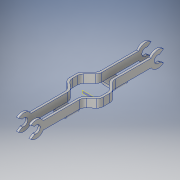
# Autodesk Inventor part: rocker
Saved by Autodesk Inventor 2018 (Build 220112000, 112)
## iProperties
Created: 2018-02-27
Part Number: rocker
Material: Aluminum 6061
Document SubType Name: Modeling
Designer: 238438
Density: 2.7 g/cm^3
Appearance: Aluminum - Flat
Author: 238438
Autodesk Inventor part; units mm, degrees
ref_plane "YZ Plane" through (0, 0, 0) normal (1, 0, 0) x (0, 1, 0)
ref_plane "XZ Plane" through (0, 0, 0) normal (0, 1, 0) x (-1, 0, 0)
ref_plane "XY Plane" through (0, 0, 0) normal (0, 0, 1) x (1, 0, 0)
sketch "Sketch1" plane through (0, 0, 0) normal (0, 1, 0) x (-1, 0, 0)
  line L0 (-1.778, -22.923) -> (-1.778, 0)
  line L1 (-0.508, -7.6359) -> (-0.508, -7.8464)
  line L2 (0, -7.62) -> (2.3608, -9.743)
  line L3 (-0.508, -7.8464) -> (1.8528, -9.9694)
  line L4 (2.3608, -10.0755) -> (2.3608, -9.743)
  line L5 (1.8528, -9.9694) -> (1.8528, -12.5094)
  line L6 (2.3608, -12.7283) -> (2.3608, -10.0755)
  line L7 (1.8528, -12.5094) -> (-0.508, -14.8702)
  line L8 (2.3608, -12.7283) -> (0, -15.1057)
  line L9 (-0.508, -15.1057) -> (-0.508, -25.2657)
  line L10 (-0.508, -25.2657) -> (0, -25.2657)
  line L11 (0, -25.2657) -> (0, -15.1057)
  line L12 (-0.508, -15.1057) -> (-0.508, -14.8702)
  line L13 (-0.508, -7.6359) -> (-0.508, 2.5241)
  line L14 (-0.508, 2.5241) -> (0, 2.5241)
  line L15 (0, 2.5241) -> (0, -7.62)
  line L16 (-5.4088, -9.9694) -> (-5.4088, -12.5094)
  line L17 (-5.9168, -12.7283) -> (-5.9168, -10.0755)
  line L18 (-3.048, -15.1057) -> (-3.048, -14.8702)
  line L19 (-5.4088, -12.5094) -> (-3.048, -14.8702)
  line L20 (-5.9168, -12.7283) -> (-3.556, -15.1057)
  line L21 (-3.048, -15.1057) -> (-3.048, -25.2657)
  line L22 (-3.048, -25.2657) -> (-3.556, -25.2657)
  line L23 (-3.556, -25.2657) -> (-3.556, -15.1057)
  line L24 (-5.9168, -10.0755) -> (-5.9168, -9.743)
  line L25 (-3.048, -7.8464) -> (-5.4088, -9.9694)
  line L26 (-3.556, -7.62) -> (-5.9168, -9.743)
  line L27 (-3.048, -7.6359) -> (-3.048, -7.8464)
  line L28 (-3.048, 2.5241) -> (-3.556, 2.5241)
  line L29 (-3.556, 2.5241) -> (-3.556, -7.62)
  line L30 (-3.048, -7.6359) -> (-3.048, 2.5241)
  point P0 (2.5714, -13.0979)
  point P1 (-0.508, -7.6086)
  point P2 (-6.1274, -13.0979)
  point P3 (-3.048, -7.6086)
  constraints: 62 end point, 18 symmetric about line, 2 coincident, 1 vertical
extrude "Extrusion1" add sketch "Sketch1" along normal blind 2.032
sketch "Sketch3" plane through (0, 0, 0) normal (0, -1, 0) x (1, 0, 0)
  line L0 (3.556, 0) -> (3.556, -6.9126) projected
  line L1 (0, -6.9126) -> (3.556, -6.9126)
  line L2 (3.556, -6.9126) -> (3.556, -3.8646)
  line L3 (3.556, -3.8646) -> (0, -3.8646)
  line L4 (0, -3.8646) -> (0, -6.9126)
  line L5 (0, -22.923) -> (0, -15.76) projected
  line L6 (3.556, -15.76) -> (3.556, -22.923) projected
  line L7 (0, -15.76) -> (3.556, -15.76)
  line L8 (3.556, -15.76) -> (3.556, -18.808)
  line L9 (3.556, -18.808) -> (0, -18.808)
  line L10 (0, -18.808) -> (0, -15.76)
  point P0 (0, 0)
  dimension "d33" = 3.048
  dimension "d34" = 3.048
  constraints: 16 end point, 4 parallel, 2 horizontal, 2 perpendicular, 2 point on line
  measures "d33" distance of L2.end L1.end
  measures "d34" distance of L7.end L8.end
extrude "Extrusion3" add sketch "Sketch3" along normal blind 0.635
fillet "Fillet4" radius 0.635 4 edges at (3.556, -0.635, -5.3886) (0, -0.635, -5.3886) (0, -0.635, -17.284) (3.556, -0.635, -17.284)
sketch "Sketch6" plane through (3.048, 0, -3.8646) normal (0, 0, 1) x (1, 0, 0)
  line L0 (-2.54, 2.032) -> (-0.0025, 2.032)
  line L1 (-0.0025, 2.032) -> (-0.0025, -3.9837)
  line L2 (-0.0025, -3.9837) -> (-2.54, -3.9837)
  line L3 (-2.54, -3.9837) -> (-2.54, 2.032)
  line L4 (-0.0025, -3.9837) -> (-2.54, -3.9837)
  line L5 (-2.54, -3.9837) -> (-2.54, 4.1191)
  line L6 (-2.54, 4.1191) -> (-0.0025, 4.1191)
  line L7 (-0.0025, 4.1191) -> (-0.0025, -3.9837)
  point P0 (-3.048, 0)
  constraints: 16 end point, 4 parallel, 2 horizontal, 2 perpendicular
extrude "Extrusion6" cut sketch "Sketch6" along normal through all
sketch "Sketch9" plane through (0.508, 0, -18.808) normal (0, 0, -1) x (-1, 0, 0)
  line L0 (0, 0) -> (0.508, 0) projected
  line L1 (0, 0) -> (-2.54, 0)
  line L2 (-2.54, 0) -> (-2.54, 7.62)
  line L3 (-2.54, 7.62) -> (0, 7.62)
  line L4 (0, 7.62) -> (0, 0)
  line L5 (-2.54, 7.62) -> (0, 7.62)
  line L6 (0, 7.62) -> (0, -7.6202)
  line L7 (0, -7.6202) -> (-2.54, -7.6202)
  line L8 (-2.54, -7.6202) -> (-2.54, 7.62)
  dimension "d50" = 2.54
  dimension "d51" = 7.62
  constraints: 16 end point, 4 parallel, 2 horizontal, 2 perpendicular, 1 point on line
  measures "d50" distance of L2.end L3.end
  measures "d51" distance of L1.end L2.end
extrude "Extrusion8" cut sketch "Sketch9" along normal through all
fillet "Fillet6" radius 1.524 16 edges at (5.9168, 1.016, -9.743) (3.556, 1.016, -7.62) (3.048, 1.016, -7.8464) (5.4088, 1.016, -9.9694) (5.4088, 1.016, -12.5094) (5.9168, 1.016, -12.7283) (3.048, 1.016, -14.8702) (3.556, 1.016, -15.1057) (-2.3608, 1.016, -12.7283) (0, 1.016, -15.1057) (0.508, 1.016, -14.8702) (-1.8528, 1.016, -12.5094) (-2.3608, 1.016, -9.743) (-1.8528, 1.016, -9.9694) (0, 1.016, -7.62) (0.508, 1.016, -7.8464)
sketch "Sketch11" plane through (0, 0, -25.2657) normal (-1, 0, 0) x (0, 0, 1)
  arc A0 (-2.3402, -0.4747) -> (-2.3402, 2.5067) centre (-1.016, 1.016) ccw
  line L0 (-1.016, 0.0802) -> (0.5328, 0.0802) construction
  line L1 (-1.016, 1.9518) -> (0.5328, 1.9518) construction
  arc A1 (-2.3402, -0.4747) -> (-2.3402, 2.5067) centre (-1.016, 1.016) ccw
  arc A2 (-1.4219, 0.1684) -> (-1.4219, 1.8636) centre (-1.016, 1.016) ccw
  line L2 (-1.4219, 1.8636) -> (-2.3402, 2.5067)
  line L3 (-1.4219, 1.8636) -> (-0.3008, 1.8636) construction
  line L4 (-1.4219, 0.1684) -> (-2.3402, -0.4747)
  line L5 (-1.4219, 0.1684) -> (-0.3008, 0.1684) construction
  point P0 (25.2657, 0)
  dimension "d66" = 3.9878
  dimension "d74" = 1.8796
  dimension "d75" = 145
  dimension "d76" = 145
  constraints: 12 end point, 6 point on circle, 4 horizontal, 3 centre point, 3 coincident, 2 equal length
  measures "d66" diameter of A0
  measures "d74" diameter of A2
  measures "d75" angle of L3 L2
  measures "d76" angle of L4 L5
extrude "Extrusion10" add sketch "Sketch11" against normal blind 3.556
sketch "Sketch12" plane through (3.048, 0, -18.808) normal (0, 0, -1) x (-1, 0, 0)
  line L0 (0, -7.62) -> (2.54, -7.62)
  line L1 (2.54, -7.62) -> (2.54, 11.139)
  line L2 (2.54, 11.139) -> (0, 11.139)
  line L3 (0, 11.139) -> (0, -7.62)
  point P0 (3.048, 0)
  constraints: 8 end point, 2 parallel, 1 horizontal, 1 perpendicular
extrude "Extrusion11" cut sketch "Sketch12" along normal through all
ref_plane "Work Plane3" through (3.048, 0, -11.3322) normal (0, 0, -1) x (-1, 0, 0)
mirror "Mirror2" about plane through (3.048, 0, -11.3322) normal (0, 0, -1) of "Extrusion10"
mirror "Mirror3" about plane through (3.048, 0, -11.3322) normal (0, 0, -1) of "Extrusion11"
body "Solid1"
